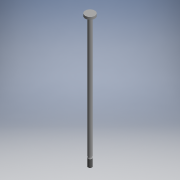
# Autodesk Inventor part: 559278 DSNU-20-200-PPS---(A---00--0-KS)
Saved by Autodesk Inventor 2017.3 (Build 213256000, 256)
## iProperties
Part Number: 559278 DSNU-20-200-PPS---(A---00--0-KS)
Material: Generic
Catalog Web Link: www.cadenas.de
Description: DSNU---(KS)-Standard cylinder
Vendor: FESTO
Document SubType Name: Modeling
Designer: partserver
Manufacturer: FESTO
Mass: 15.2977 g
Surface Area: 78.2668 cm^2
Volume: 15.2977 cm^3
Density: 1 g/cm^3
Appearance: PSOLRGB-192-192-192
Category: PARTsolutions
Company: FESTO
Title: 559278 DSNU-20-200-PPS
Author: Cadenas PARTsolutions
Comments: Standard cylinder
PSOL_IDENT_0: {$CADENAS_DATA\23d-libs\festo\parts\d\dsnu\parts\dsnu_metric_ks.prj},260 {VTYP=3D},{NB=559278 DSNU-2
PSOL_IDENT_1: 0-200-PPS---(A---00--0-KS)},{LINA=559278 DSNU-20-200-PPS},{NN=DSNU---(KS)},{DATE=25.01.2021 09:43:10
PSOL_IDENT_2: },{GEOMDATE=06.03.2020 09:03:14},{VERSION=},{LINEID=50},{WBVAR=TNR,HUB,DA,PE,ZD,VS,KA,K2A,K6,K3,K5,K
PSOL_IDENT_3: 8,KP},{WBNUMERIC=HUB,K2A,K6,K8}  {NB=559278 DSNU-20-200-PPS---(A---00--0-KS)},{LINA=559278 DSNU-20-2
PSOL_IDENT_4: 00-PPS},{KT=DUMMY},{TNR=559278},{TYP=DSNU-20},{DSNU=METRIC},{KDM=20},{HUB=200},{DA=PPS},{DA1='P','PP
PSOL_IDENT_5: V','PPS'},{PE=A},{ZD=-},{VS=-},{VSALG='-','Q'},{KA=-},{KAALG='-','S2'},{K2A=0},{K6=0},{K3=-},{K31='-'
PSOL_IDENT_6: ,'K3'},{K5=-},{K51='-'},{K8=0},{KP=-},{KPALG='-','KP'},{A1=25},{A2=110},{A3=8},{A4=47.0},{AB=22},{AM=
PSOL_IDENT_7: 20},{B=22},{BB=3},{BE=M22x1,5},{BENDM=22.000},{BEKDM=20.160},{BEP=1.500},{BS=5.5},{B1=40},{B2=0},{B3=
PSOL_IDENT_8: 0},{B4=0},{B5=22.4},{B6=10},{B7=0},{CD=8},{D=27},{D1=22},{D2=8},{D3=21.3},{D4=7.0},{D5=21.7},{D6=0},
PSOL_IDENT_9: {D7=0},{EE=G1/8},{EENDM=9.728},{EEKDM=8.566},{EW=16},{F=31},{FF=M5},{FFNDM=5.000},{FFKDM=4.019},{F1=
PSOL_IDENT_10: 0},{H=28},{H1=0},{KK=M8},{KKNDM=8.000},{KKKDM=0.000},{KKP=1.250},{K1=M4},{K1NDM=4.000},{K1KDM=3.141}
PSOL_IDENT_11: ,{K2=0.0},{KV=32},{KW=11},{L=12},{LH=7.5},{LK=14.5},{L1=112},{L2=68},{L3=8.2},{L4=20.0},{L5=18},{L6=
PSOL_IDENT_12: 44},{L7=24},{L8=16.0},{L9=29.0},{L10=82},{L11=92},{L12=66.5},{L13=116.0},{ST=5.5},{SW=7},{T=12},{WH=
PSOL_IDENT_13: 24},{X=2.0},{XC=95},{K1KP=36},{K2KP=M5},{K2KPNDM=5.000},{K3KP=11},{K4KP=18.0},{K5KP=62.5},{K6KP=4.2}
PSOL_IDENT_14: ,{K7KP=20},{K8KP=27.0},{K9KP=13.0},{K10KP=4.5},{K11KP=20},{K12KP=M5},{K12KPNDM=5.000},{K13KP=47},{ZR
PSOL_IDENT_15: START=36},{MHL=30.000},{ZRL=36},{C=14.500},{WHX=10.000},{LD1=20.000},{LD2=19.700},{AD1=11.000},{AD2=
PSOL_IDENT_16: 8.000},{AD3=16.000},{AD4=8.000},{AD5=22.200},{MH1=9.000},{MH2=4.200},{MH3=13.000},{KP1=29.000},{KP2=
PSOL_IDENT_17: 14.500},{KP3=12.000},{KP4=20.000},{KP5=26.000},{KPC=18.000},{KPF=3.000},{KPG=17.500},{KPH=62.000},{K
PSOL_IDENT_18: PJ=19.500},{KPK=17.000},{KPL=4.500},{KPR3=1.000},{KPR=19.000},{KPS=16.000},{MLD1=35.000},{MLD2=30.00
PSOL_IDENT_19: 0},{MLD3=4.000},{MLL1=12.000},{KL1=54.3},{KKC=6.4},{KKD=1.5},{KKF=0.6},{SWL=3.000},{K3L=4.300},{HUB1=
PSOL_IDENT_20: 200},{FDTXF31=4.000},{FDTB31=4.000}
NB: 559278 DSNU-20-200-PPS---(A---00--0-KS)
NN: DSNU---(KS)
NT: Standard cylinder
NBSYN: $TNR. $TYP.-$HUB1.-$DA.---($PE.$ZD.$VS.$KA.$K2A.$K6.$K3.$K5.$K8.$KP.KS)
LINA: 559278 DSNU-20-200-PPS
CATALOG: Festo
TNR: 559278
TYP: DSNU-20
DSNU: METRIC
KDM: 20
HUB: 200
DA: PPS
DA1: 'P','PPV','PPS'
PE: A
ZD: -
VS: -
KA: -
K2A: 0
K6: 0
K3: -
K31: '-','K3'
K5: -
K51: '-'
K8: 0
KP: -
A1: 25
A2: 110
A3: 8
A4: 47
AB: 22
AM: 20
B: 22
BB: 3
BE: M22x1,5
BENDM: 22
BEKDM: 20.16
BEP: 1.5
BS: 5.5
B1: 40
B2: 0
B3: 0
B4: 0
B5: 22.4
B6: 10
B7: 0
CD: 8
D: 27
D1: 22
D2: 8
D3: 21.3
D4: 7
D5: 21.7
D6: 0
D7: 0
EE: G1/8
EENDM: 9.728
EEKDM: 8.566
EW: 16
F: 31
FF: M5
FFNDM: 5
FFKDM: 4.019
F1: 0
H: 28
H1: 0
KK: M8
KKNDM: 8
KKKDM: 0
KKP: 1.25
K1: M4
K1NDM: 4
K1KDM: 3.141
K2: 0
KV: 32
KW: 11
L: 12
LH: 7.5
LK: 14.5
L3: 8.2
L4: 20
L5: 18
L6: 44
L7: 24
L8: 16
L9: 29
L13: 116
ST: 5.5
SW: 7
T: 12
X: 2
K1KP: 36
K2KP: M5
K2KPNDM: 5
K3KP: 11
K4KP: 18
K5KP: 62.5
K6KP: 4.2
K7KP: 20
K8KP: 27
K9KP: 13
K10KP: 4.5
K11KP: 20
K12KP: M5
K12KPNDM: 5
K13KP: 47
MHL: 30
C: 14.5
WHX: 10
LD1: 20
LD2: 19.7
AD1: 11
AD2: 8
AD3: 16
AD4: 8
AD5: 22.2
MH1: 9
MH2: 4.2
MH3: 13
KP1: 29
KP2: 14.5
KP3: 12
KP4: 20
KP5: 26
KPC: 18
KPF: 3
KPG: 17.5
KPH: 62
KPJ: 19.5
KPK: 17
KPL: 4.5
KPR3: 1
KPR: 19
KPS: 16
MLD1: 35
MLD2: 30
MLD3: 4
MLL1: 12
SWL: 3
K3L: 4.3
FDTXF31: 4
FDTB31: 4
SUPPLIER: FESTO
ARTICLENO: 559278 DSNU-20-200-PPS---(A---00--0-KS)
BOMINFO: 559278 DSNU-20-200-PPS
CREATOR: CADENAS GmbH
Autodesk Inventor part; units mm, degrees
sketch "Sketch_2" plane through (0, 0, 0) normal (1, 0, 0) x (0, 1, 0)
  line L0 (0, -255.3) -> (0, 4)
  line L1 (0, 4) -> (4, 4)
  line L2 (4, 4) -> (4, -250.3)
  line L3 (4, -250.3) -> (10, -250.3)
  line L4 (10, -250.3) -> (10, -255.3)
  line L5 (10, -255.3) -> (0, -255.3)
  line L6 (0, -255.3) -> (0, 4)
  constraints: 14 end point
revolve "Revolution1" add sketch "Sketch_2" angle 360 about axis through (0, 0, -255.3) along (0, 0, -1)
sketch "Sketch_6" plane through (0, 0, 0) normal (1, 0, 0) x (0, 1, 0)
  line L0 (0, 3) -> (0, 24)
  line L1 (0, 24) -> (3.233, 24)
  line L2 (3.233, 24) -> (4, 23.233)
  line L3 (4, 23.233) -> (4, 7.698)
  line L4 (4, 7.698) -> (3.2362, 5.5994)
  arc A0 (3.2362, 5.5994) -> (3.2, 5.3942) centre (3.8, 5.3942) ccw
  line L5 (3.2, 5.3942) -> (3.2, 4.6)
  arc A1 (3.2, 4.6) -> (3.8, 4) centre (3.8, 4.6) ccw
  line L6 (3.8, 4) -> (4, 4)
  line L7 (4, 4) -> (4, 3)
  line L8 (4, 3) -> (0, 3)
  line L9 (0, 3) -> (0, 24)
  constraints: 20 end point, 4 point on circle, 2 centre point
revolve "Revolution2" add sketch "Sketch_6" angle 360 about axis through (0, 0, 3) along (0, 0, -1)
thread "Thread1" size "M8x1.25" class "6g" standard "ISO Metric profile" full length
sketch "Sketch_7" plane through (0, 0, 1) normal (0, 0, 1) x (1, 0, 0)
  line L0 (-7, 14) -> (-7, -7)
  line L1 (-7, -7) -> (-3.5, -7)
  line L2 (-3.5, -7) -> (-3.5, 7)
  line L3 (-3.5, 7) -> (3.5, 7)
  line L4 (3.5, 7) -> (3.5, -7)
  line L5 (3.5, -7) -> (7, -7)
  line L6 (7, -7) -> (7, 14)
  line L7 (7, 14) -> (-7, 14)
  constraints: 16 end point
extrude "Extrusion1" cut sketch "Sketch_7" along normal blind 4
ref_plane "FDT_KSAUFSATZ_XY" through (0, 0, 12) normal (0, 0, 1) x (-1, 0, 0)
ref_plane "FDT_KSAUFSATZ_YZ" through (0, 0, 12) normal (-1, 0, 0) x (0, -1, 0)
ref_plane "FDT_KSAUFSATZ_ZX" through (0, 0, 12) normal (0, -1, 0) x (0, 0, 1)
ref_plane "FDT_NUT_XY" through (0, 0, 12) normal (0, 0, 1) x (-1, 0, 0)
ref_plane "FDT_NUT_YZ" through (0, 0, 12) normal (-1, 0, 0) x (0, -1, 0)
ref_plane "FDT_NUT_ZX" through (0, 0, 12) normal (0, -1, 0) x (0, 0, 1)
ref_plane "KS_XY" through (0, 0, 0) normal (0, 0, -1) x (1, 0, 0)
ref_plane "KS_YZ" through (0, 0, 0) normal (1, 0, 0) x (0, -1, 0)
ref_plane "KS_ZX" through (0, 0, 0) normal (0, -1, 0) x (0, 0, -1)
ref_plane "NUT1_XY" through (0, 0, 20) normal (0, 0, 1) x (1, 0, 0)
ref_plane "NUT1_YZ" through (0, 0, 20) normal (1, 0, 0) x (0, 1, 0)
ref_plane "NUT1_ZX" through (0, 0, 20) normal (0, 1, 0) x (0, 0, 1)
body "Solid1"
